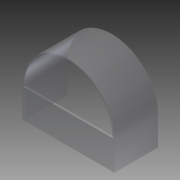
# Autodesk Inventor part: Bucket Flap
Saved by Autodesk Inventor 2015 (Build 190159000, 159)
## iProperties
Created: 2015-03-01
Part Number: Bucket Flap
Material: Polycarbonate, Clear
Document SubType Name: Modeling
Designer: patel_000
Density: 1.2 g/cm^3
Appearance: Polycarbonate - Clear
Author: patel_000
Autodesk Inventor part; units mm, degrees
ref_plane "YZ Plane" through (0, 0, 0) normal (1, 0, 0) x (0, 1, 0)
ref_plane "XZ Plane" through (0, 0, 0) normal (0, 1, 0) x (-1, 0, 0)
ref_plane "XY Plane" through (0, 0, 0) normal (0, 0, 1) x (1, 0, 0)
sketch "Sketch1" plane through (0, 0, 0) normal (0, 0, 1) x (1, 0, 0)
  line L0 (59.7408, 0) -> (59.7408, -50.8)
  line L1 (-101.6, -50.8) -> (-101.6, 0)
  arc A0 (59.7408, 0) -> (-101.6, 0) centre (-20.9296, 0) ccw
  arc A1 (56.5658, 0) -> (-98.425, 0) centre (-20.9296, 0) ccw
  line L2 (-98.425, 0) -> (-98.425, -50.8)
  line L3 (56.5658, -50.8) -> (56.5658, 0)
  line L4 (-101.6, 0) -> (-98.425, 0)
  line L5 (56.5658, 0) -> (59.7408, 0)
  line L6 (-101.6, 0) -> (-98.425, 0)
  line L7 (56.5658, 0) -> (59.7408, 0)
  line L8 (59.7408, -50.8) -> (56.5658, -50.8)
  line L9 (-98.425, -50.8) -> (-101.6, -50.8)
  point P0 (0, 0)
  dimension "d5" = 161.3408
  dimension "d6" = 50.8
  dimension "d7" = 3.175
  dimension "d8" = 3.175
  constraints: 20 end point, 6 perpendicular, 5 parallel, 4 horizontal, 4 point on circle, 2 centre point, 2 tangent
  measures "d5" distance of L0.end L1.start
  measures "d6" distance of L0.start L0.end
  measures "d7" distance of L1.end L2.start
  measures "d8" distance of L0.start L3.end
extrude "Extrusion1" add sketch "Sketch1" along normal blind 76.2
sketch "Sketch2" plane through (0, 0, 76.2) normal (0, 0, 1) x (1, 0, 0)
  line L0 (-101.6, 0) -> (59.7408, 0)
  line L1 (59.7408, 0) -> (59.7408, -50.8)
  line L2 (59.7408, -50.8) -> (-101.6, -50.8)
  line L3 (-101.6, -50.8) -> (-101.6, 0)
  point P0 (0, 0)
  constraints: 8 end point, 2 parallel, 1 horizontal, 1 perpendicular
extrude "Extrusion2" add sketch "Sketch2" against normal blind 3.175
body "Solid1"
